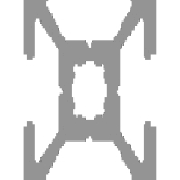
# Autodesk Inventor part: 20x20_bosch profile
Saved by Autodesk Inventor 2021.3 (Build 253353000, 353)
## iProperties
Created: 2024-01-11
Part Number: 20x20_bosch profile
Material: Aluminum 6061
Document SubType Name: Modeling
Designer: nxf77172
Language: en-US
Size Designation: (Unnamed 1)
Categories: <MemberInstance><Categories><Category DisplayName="Structural Shapes" InternalName="089c4875-fa83-4c05-b084-43b9cc11f5ed" Mnemonic="GRDR"><CategoryParameter DisplayName="Mass per Length Unit" InternalName="0bb95a10-148f-4027-a459-38d7b056702a" Mnemonic="shpmass"/><CategoryParameter DisplayName="Section Area" InternalName="1ff91680-64b0-4202-b9a3-7fd3f94bba3b" Mnemonic="secarea"/><CategoryParameter DisplayName="Radius of Gyration (x)" InternalName="25778675-03e9-40c1-b6a8-4a9ed693320d" Mnemonic="gyrradx"/><CategoryParameter DisplayName="Torsional Rigidity Modulus" InternalName="26c1ec35-5026-4c63-ad0a-751cf684a536" Mnemonic="torrigmod"/><CategoryParameter DisplayName="Distance of the Center of Gravity X-X" InternalName="26c9bdb8-9c79-4b4f-a92e-8e197583c9c4" Mnemonic="grcendistX"/><CategoryParameter DisplayName="Legacy Member ID" InternalName="340afe4f-75d7-48d3-ab7d-943f3c3da468" Mnemonic="LegacyMemberID"/><CategoryParameter DisplayName="Base Length" InternalName="42e34263-8f20-4d0e-ad48-bf1385b87c24" Mnemonic="shplen"/><CategoryParameter DisplayName="Moment of Inertia (y)" InternalName="4b9f58ea-bced-460e-81ea-3d29ca5a49e3" Mnemonic="inermomy"/><CategoryParameter DisplayName="Moment of Inertia (x)" InternalName="4cd780bc-73d7-43ac-917a-579e5cbd684d" Mnemonic="inermomx"/><CategoryParameter DisplayName="Custom Base Point" InternalName="4f1d1b73-316d-484b-a3df-9cbabb16eb77" Mnemonic="shpBasePoint"/><CategoryParameter DisplayName="Shape Height" InternalName="50274e7d-5ac0-4796-92cb-c59e54983c67" Mnemonic="shpheig"/><CategoryParameter DisplayName="Section Module (y)" InternalName="59eaa5e9-d227-48dc-b6c1-6920f96e0f95" Mnemonic="secmody"/><CategoryParameter DisplayName="Section Designation" InternalName="5a64d034-428d-49c8-ba32-7619764de20f" Mnemonic="shpdes"/><CategoryParameter DisplayName="Section Module (x)" InternalName="72cfad18-cf51-4ed4-aaa7-c6b224f8419f" Mnemonic="secmodx"/><CategoryParameter DisplayName="Torsional Section Modulus" InternalName="7c55a8dc-8844-49f9-a867-cc677b30ec9a" Mnemonic="torsecmod"/><CategoryParameter DisplayName="Shape Width" InternalName="7c717d54-a18f-4666-b4d4-573cce22c62c" Mnemonic="shpwdth"/><CategoryParameter DisplayName="Second Shape Thickness" InternalName="9251a8e1-85fd-4e47-af99-afdb762317d9" Mnemonic="shpthick2"/><CategoryParameter DisplayName="FG Authored" InternalName="9c666724-f362-4ea7-ac62-f6a007de5c69" Mnemonic="shpFGAuto"/><CategoryParameter DisplayName="Distance of the Center of Gravity Y-Y" InternalName="bcc4fb17-7af4-436a-8f8c-d0aa3b0248c5" Mnemonic="grcendistY"/><CategoryParameter DisplayName="Radius of Gyration (y)" InternalName="bfa18ebe-1636-4dbe-8d42-b263e0b73184" Mnemonic="gyrrady"/><CategoryParameter DisplayName="Shape Thickness" InternalName="d109cf76-8eb4-42fc-9800-4409734adc67" Mnemonic="shpthick"/><CategoryParameter DisplayName="Coefficient of Shear Displacement" InternalName="de4c90c6-aaa8-468f-a335-6737b311b5d3" Mnemonic="shdispc"/><Category DisplayName="Other" InternalName="f02205ff-2390-476f-921c-0b3185f88e84" Mnemonic="OTHSHP"><CategoryParameter DisplayName="Moment of Inertia (y)" InternalName="044c654e-f649-48ac-84cc-650a29ae31ca" Mnemonic="inermomy"/><CategoryParameter DisplayName="Shape Thickness" InternalName="12b1a788-9233-48fd-a933-2df8ff42b15f" Mnemonic="shpthick"/><CategoryParameter DisplayName="Mass per Length Unit" InternalName="2fd289d6-9394-4d2d-97e6-6659d7d4551d" Mnemonic="shpmass"/><CategoryParameter DisplayName="Radius of Gyration (y)" InternalName="743e1dfe-1bba-408b-b985-cf752b207386" Mnemonic="gyrrady"/><CategoryParameter DisplayName="Section Module (y)" InternalName="88b8bff9-a616-4028-93d5-ed4f79680d13" Mnemonic="secmody"/><CategoryParameter DisplayName="Section Area" InternalName="c46ecdf8-b6eb-4db9-8b25-30258930c1e3" Mnemonic="secarea"/><CategoryParameter DisplayName="Section Module (x)" InternalName="cac70804-9d39-43bb-be17-56ea1f39a6c2" Mnemonic="secmodx"/><CategoryParameter DisplayName="Moment of Inertia (x)" InternalName="ec6737bc-264f-43ed-b0bd-f6d410c2718d" Mnemonic="inermomx"/><CategoryParameter DisplayName="Radius of Gyration (x)" InternalName="ee72c61e-565e-4fd6-b448-66e1e1abcb7e" Mnemonic="gyrradx"/></Category></Category><Category DisplayName="DataType" InternalName="23b78d0f-2648-40c6-8793-ca6db495c9e8" Mnemonic="DATATYPE"><CategoryParameter DisplayName="DisplayName" InternalName="05415f3d-3907-474b-a020-eb9d644f4cf3" Mnemonic="DISPLAYNAME"/><CategoryParameter DisplayName="Standard" InternalName="0c0a119c-1e12-4c84-803f-101930972f5e" Mnemonic="STANDARD"/><CategoryParameter DisplayName="Description" InternalName="13903e3d-64b1-4950-80da-f627842ea37f" Mnemonic="DESCRIPTION"/><CategoryParameter DisplayName="Designation" InternalName="2675968c-4ce5-49e0-a4f5-552d29089031" Mnemonic="DESIGNATION"/><CategoryParameter DisplayName="Default Row" InternalName="2af9ec52-faaa-4026-b378-f9fa4afca842" Mnemonic="DEFAULTROW"/><CategoryParameter DisplayName="Folder Name" InternalName="3f06958e-8713-4116-9be7-ed6184ecc97b" Mnemonic="FOLDERNAME"/><CategoryParameter DisplayName="Revision Guid" InternalName="45a75005-10b1-4dfc-8d6d-dfe629f0b93c" Mnemonic="REVISIONGUID"/><CategoryParameter DisplayName="FileName" InternalName="8b46a4cc-9585-4fed-90c3-899f57e09a73" Mnemonic="FILENAME"/><CategoryParameter DisplayName="StdsOrg" InternalName="8f5914e1-4693-403f-8ab5-d37768198c9d" Mnemonic="STDSORG"/><CategoryParameter DisplayName="Family Version" InternalName="914462f6-6e19-4b14-ba84-155b9680b1d0" Mnemonic="FAMILYREVISION"/><CategoryParameter DisplayName="Standard Revision" InternalName="91d5a463-65c2-4fde-b823-3b7fea5e8e17" Mnemonic="STANDARDREVISION"/><CategoryParameter DisplayName="Member Revision" InternalName="a65d44b9-392f-4f4f-857b-e4b3d54996fe" Mnemonic="MEMBERREVISION"/><CategoryParameter DisplayName="ClipFormat" InternalName="bc51e27b-3422-4e78-93ef-cec197ddf230" Mnemonic="CLIPFORMAT"/><CategoryParameter DisplayName="Manufacturer" InternalName="cd6c7a72-a28a-4e50-99a9-2c7f4e13e5ad" Mnemonic="MANUFACTURER"/><CategoryParameter DisplayName="InternalName" InternalName="cf1d0246-76d9-4b4a-8305-fa0409afb5c1" Mnemonic="INTERNALNAME"/><CategoryParameter DisplayName="IsMetric" InternalName="e2385c5b-1ea4-4823-96a8-8de651266ec3" Mnemonic="ISMETRIC"/><Category DisplayName="Part" InternalName="c0e0b642-3bcb-4cc8-9e80-f96d35c4afa4" Mnemonic="PART"><CategoryParameter DisplayName="Part Number" InternalName="016b6077-bfbe-49bd-92c9-d8d59c39c941" Mnemonic="PARTNUMBER"/><CategoryParameter DisplayName="Stock Number" InternalName="4dba7c1c-e26c-444e-836c-b08b433409a8" Mnemonic="STOCKNUMBER"/><CategoryParameter DisplayName="Material Key" InternalName="5c9a8adb-dd2b-4535-b97f-0a94a95fe41f" Mnemonic="MATERIALKEY"/><CategoryParameter DisplayName="Material" InternalName="818a152a-d3c3-49ca-80ee-df7d91421b8e" Mnemonic="MATERIAL"/></Category></Category></Categories><FamilyTemplate Id="20x20_bosch profile"><FamilyTemplateParameters><FamilyTemplateParameter ObjectType="kUserParameterObject" ValueType="xs:double" Id="12" ObjectReferenceKey="Length"/><FamilyTemplateParameter ObjectType="kPartComponentDefinitionObject" ValueType="xs:string" Id="23" SubObjectId="Material"/><FamilyTemplateParameter ObjectType="kPropertyObject" ValueType="xs:string" Id="26" ObjectReferenceKey="{32853F0F-3444-11d1-9E93-0060B03C1CA6}" SubObjectId="5"/><FamilyTemplateParameter ObjectType="kPropertyObject" ValueType="xs:string" Id="27" ObjectReferenceKey="{32853F0F-3444-11d1-9E93-0060B03C1CA6}" SubObjectId="52"/></FamilyTemplateParameters></FamilyTemplate><CategoryParameterMap><ParamToTemplateMap><ParamToTemplate CategoryParameter="//CategoryParameter[@InternalName='cf1d0246-76d9-4b4a-8305-fa0409afb5c1']" ConstantValue="27b4ad4a-2417-46ba-b811-a387dd64a500"/><ParamToTemplate CategoryParameter="//CategoryParameter[@InternalName='45a75005-10b1-4dfc-8d6d-dfe629f0b93c']" ConstantValue="f0b9e895-ce42-4fe4-8826-9398c456ece3"/><ParamToTemplate CategoryParameter="//CategoryParameter[@InternalName='3f06958e-8713-4116-9be7-ed6184ecc97b']" ConstantValue="20x20_bosch profile"/><ParamToTemplate CategoryParameter="//CategoryParameter[@InternalName='8f5914e1-4693-403f-8ab5-d37768198c9d']" TemplateParameter="17"/><ParamToTemplate CategoryParameter="//CategoryParameter[@InternalName='0c0a119c-1e12-4c84-803f-101930972f5e']" TemplateParameter="18"/><ParamToTemplate CategoryParameter="//CategoryParameter[@InternalName='91d5a463-65c2-4fde-b823-3b7fea5e8e17']" TemplateParameter="19"/><ParamToTemplate CategoryParameter="//CategoryParameter[@InternalName='cd6c7a72-a28a-4e50-99a9-2c7f4e13e5ad']" TemplateParameter="20"/><ParamToTemplate CategoryParameter="//CategoryParameter[@InternalName='13903e3d-64b1-4950-80da-f627842ea37f']" TemplateParameter="22"/><ParamToTemplate CategoryParameter="//CategoryParameter[@InternalName='05415f3d-3907-474b-a020-eb9d644f4cf3']" ConstantValue="20x20_bosch profile"/><ParamToTemplate CategoryParameter="//CategoryParameter[@InternalName='914462f6-6e19-4b14-ba84-155b9680b1d0']" ConstantValue="11"/><ParamToTemplate CategoryParameter="//CategoryParameter[@InternalName='bc51e27b-3422-4e78-93ef-cec197ddf230']" ConstantValue="CF_INVENTOR.STDPARTS"/><ParamToTemplate CategoryParameter="//CategoryParameter[@InternalName='e2385c5b-1ea4-4823-96a8-8de651266ec3']" ConstantValue="true"/><ParamToTemplate CategoryParameter="//CategoryParameter[@InternalName='2af9ec52-faaa-4026-b378-f9fa4afca842']" ConstantValue="1"/><ParamToTemplate CategoryParameter="//CategoryParameter[@InternalName='9c666724-f362-4ea7-ac62-f6a007de5c69']" ConstantValue="1"/><ParamToTemplate CategoryParameter="//CategoryParameter[@InternalName='8b46a4cc-9585-4fed-90c3-899f57e09a73']" ConstantValue="Aluminum 6061-1"/><ParamToTemplate CategoryParameter="//CategoryParameter[@InternalName='a65d44b9-392f-4f4f-857b-e4b3d54996fe']" ConstantValue="857d2c95-77cc-4b79-b9be-8e574b0f7ae4"/><ParamToTemplate CategoryParameter="//CategoryParameter[@InternalName='a65d44b9-392f-4f4f-857b-e4b3d54996fe']" ConstantValue="857d2c95-77cc-4b79-b9be-8e574b0f7ae4"/><ParamToTemplate CategoryParameter="//CategoryParameter[@InternalName='2675968c-4ce5-49e0-a4f5-552d29089031']" TemplateParameter="27"/><ParamToTemplate CategoryParameter="//CategoryParameter[@InternalName='42e34263-8f20-4d0e-ad48-bf1385b87c24']" TemplateParameter="12"/><ParamToTemplate CategoryParameter="//CategoryParameter[@InternalName='818a152a-d3c3-49ca-80ee-df7d91421b8e']" TemplateParameter="23"/><ParamToTemplate CategoryParameter="//CategoryParameter[@InternalName='016b6077-bfbe-49bd-92c9-d8d59c39c941']" TemplateParameter="26"/></ParamToTemplateMap></CategoryParameterMap></MemberInstance>
Mass: 0.435942 g
Surface Area: 5.07764 cm^2
Volume: 0.16146 cm^3
Density: 2.7 g/cm^3
Appearance: Aluminum - Flat
IsCustomPart: 1
Length: 200.000 mm
G_L: 200.000 mm
G_W: 20.000 mm
G_H: 20.000 mm
_CCFamilyDisplayName: 20x20_bosch profile
_FrameMemberDoc: Frame Member File
_Version: 15.0.0
_GetPNFromCC: 1
Author: nxf77172
Autodesk Inventor part; units mm, degrees
ref_plane "YZ Plane" through (0, 0, 0) normal (1, 0, 0) x (0, 1, 0)
ref_plane "Start Plane" through (0, 0, 0) normal (0, 1, 0) x (-1, 0, 0)
ref_plane "End Plane" through (0, 200, 0) normal (0, 1, 0) x (-1, 0, 0)
sketch "Sketch" plane through (0, 0, 0) normal (0, 1, 0) x (-1, 0, 0)
  line L0 (8.5, 10) -> (3.5, 10)
  line L1 (4.5, 0.5) -> (4.5, 3.2322)
  line L2 (3.2322, 4.5) -> (0.5, 4.5)
  line L3 (3, 9.5) -> (3, 9)
  line L4 (3.5, 8.5) -> (6.2322, 8.5)
  line L5 (8.5, 6.2322) -> (8.5, 3.5)
  line L6 (9, 3) -> (9.5, 3)
  line L7 (6.5858, 7.6464) -> (3.5858, 4.6464)
  line L8 (7.6464, 6.5858) -> (4.6464, 3.5858)
  line L9 (10, 10) -> (0, 0) construction
  line L10 (0.5, 4.5) -> (0, 4)
  line L11 (3, 9.5) -> (3.5, 9.5)
  line L12 (3.5, 9.5) -> (3.5, 10)
  line L13 (9.5, 3) -> (9.5, 3.5)
  line L14 (9.5, 3.5) -> (10, 3.5)
  line L15 (10, 3.5) -> (10, 10)
  line L16 (0, 0) -> (10, 0) construction
  line L17 (10, 0) -> (10, 8.5) construction
  line L18 (0, 0) -> (0, 10) construction
  line L19 (0, 10) -> (10, 10) construction
  line L20 (4.5, 0.5) -> (4, 0)
  arc A0 (10, 8.5) -> (8.5, 10) centre (8.5, 8.5) ccw
  arc A1 (3, 9) -> (3.5, 8.5) centre (3.5, 9) ccw
  arc A2 (6.5858, 7.6464) -> (6.2322, 8.5) centre (6.2322, 8) ccw
  arc A3 (8.5, 6.2322) -> (7.6464, 6.5858) centre (8, 6.2322) ccw
  arc A4 (8.5, 3.5) -> (9, 3) centre (9, 3.5) ccw
  arc A5 (4.6464, 3.5858) -> (4.5, 3.2322) centre (5, 3.2322) ccw
  arc A6 (3.2322, 4.5) -> (3.5858, 4.6464) centre (3.2322, 5) ccw
  line L21 (2.2657, 2.2657) -> (1.9121, 2.6192)
  line L22 (2.2657, 2.2657) -> (2.6192, 1.9121)
  line L23 (1.9121, 2.6192) -> (1.5586, 2.2657)
  line L24 (2.6192, 1.9121) -> (2.2657, 1.5586)
  arc A7 (2.75, 0) -> (2.2657, 1.5586) centre (0, 0) ccw
  arc A8 (1.5586, 2.2657) -> (0, 2.75) centre (0, 0) ccw
  line L25 (0, 0) -> (10, 0) construction
  line L26 (10, -10) -> (0, 0) construction
  line L27 (0, 0) -> (0, -10) construction
  line L28 (0, -10) -> (8.5, -10) construction
  line L29 (0.5, -4.5) -> (3.2322, -4.5)
  line L30 (0.5, -4.5) -> (0, -4)
  line L31 (1.9121, -2.6192) -> (1.5586, -2.2657)
  arc A9 (0, -2.75) -> (1.5586, -2.2657) centre (0, 0) ccw
  arc A10 (7.6464, -6.5858) -> (8.5, -6.2322) centre (8, -6.2322) ccw
  line L32 (8.5, -3.5) -> (8.5, -6.2322)
  line L33 (10, -8.5) -> (10, -3.5)
  line L34 (3.5, -10) -> (10, -10)
  line L35 (6.5858, -7.6464) -> (3.5858, -4.6464)
  line L36 (7.6464, -6.5858) -> (4.6464, -3.5858)
  line L37 (10, 0) -> (10, -10) construction
  line L38 (4.5, -3.2322) -> (4.5, -0.5)
  arc A11 (8.5, -10) -> (10, -8.5) centre (8.5, -8.5) ccw
  line L39 (6.2322, -8.5) -> (3.5, -8.5)
  arc A12 (3.5, -8.5) -> (3, -9) centre (3.5, -9) ccw
  arc A13 (6.2322, -8.5) -> (6.5858, -7.6464) centre (6.2322, -8) ccw
  line L40 (3, -9.5) -> (3.5, -9.5)
  line L41 (3.5, -9.5) -> (3.5, -10)
  line L42 (9.5, -3) -> (9, -3)
  line L43 (4.5, -0.5) -> (4, 0)
  line L44 (9.5, -3) -> (9.5, -3.5)
  line L45 (9.5, -3.5) -> (10, -3.5)
  arc A14 (4.5, -3.2322) -> (4.6464, -3.5858) centre (5, -3.2322) ccw
  arc A15 (9, -3) -> (8.5, -3.5) centre (9, -3.5) ccw
  arc A16 (3.5858, -4.6464) -> (3.2322, -4.5) centre (3.2322, -5) ccw
  line L46 (3, -9) -> (3, -9.5)
  line L47 (2.2657, -2.2657) -> (2.6192, -1.9121)
  line L48 (2.2657, -2.2657) -> (1.9121, -2.6192)
  line L49 (2.6192, -1.9121) -> (2.2657, -1.5586)
  arc A17 (2.2657, -1.5586) -> (2.75, 0) centre (0, 0) ccw
  line L50 (0, 0) -> (0, -10) construction
  line L51 (-10, -10) -> (0, 0) construction
  line L52 (0, 0) -> (-10, 0) construction
  line L53 (-10, 0) -> (-10, -8.5) construction
  line L54 (-4.5, -0.5) -> (-4.5, -3.2322)
  line L55 (-4.5, -0.5) -> (-4, 0)
  line L56 (-2.6192, -1.9121) -> (-2.2657, -1.5586)
  arc A18 (-2.75, 0) -> (-2.2657, -1.5586) centre (0, 0) ccw
  arc A19 (-6.5858, -7.6464) -> (-6.2322, -8.5) centre (-6.2322, -8) ccw
  line L57 (-3.5, -8.5) -> (-6.2322, -8.5)
  line L58 (-8.5, -10) -> (-3.5, -10)
  line L59 (-10, -3.5) -> (-10, -10)
  line L60 (-7.6464, -6.5858) -> (-4.6464, -3.5858)
  line L61 (-6.5858, -7.6464) -> (-3.5858, -4.6464)
  line L62 (0, -10) -> (-10, -10) construction
  line L63 (-3.2322, -4.5) -> (-0.5, -4.5)
  arc A20 (-10, -8.5) -> (-8.5, -10) centre (-8.5, -8.5) ccw
  line L64 (-8.5, -6.2322) -> (-8.5, -3.5)
  arc A21 (-8.5, -3.5) -> (-9, -3) centre (-9, -3.5) ccw
  arc A22 (-8.5, -6.2322) -> (-7.6464, -6.5858) centre (-8, -6.2322) ccw
  line L65 (-9.5, -3) -> (-9.5, -3.5)
  line L66 (-9.5, -3.5) -> (-10, -3.5)
  line L67 (-3, -9.5) -> (-3, -9)
  line L68 (-0.5, -4.5) -> (0, -4)
  line L69 (-3, -9.5) -> (-3.5, -9.5)
  line L70 (-3.5, -9.5) -> (-3.5, -10)
  arc A23 (-3.2322, -4.5) -> (-3.5858, -4.6464) centre (-3.2322, -5) ccw
  arc A24 (-3, -9) -> (-3.5, -8.5) centre (-3.5, -9) ccw
  arc A25 (-4.6464, -3.5858) -> (-4.5, -3.2322) centre (-5, -3.2322) ccw
  line L71 (-9, -3) -> (-9.5, -3)
  line L72 (-2.2657, -2.2657) -> (-1.9121, -2.6192)
  line L73 (-2.2657, -2.2657) -> (-2.6192, -1.9121)
  line L74 (-1.9121, -2.6192) -> (-1.5586, -2.2657)
  arc A26 (-1.5586, -2.2657) -> (0, -2.75) centre (0, 0) ccw
  line L75 (0, 0) -> (-10, 0) construction
  line L76 (-10, 10) -> (0, 0) construction
  line L77 (0, 0) -> (0, 10) construction
  line L78 (0, 10) -> (-8.5, 10) construction
  line L79 (-0.5, 4.5) -> (-3.2322, 4.5)
  line L80 (-0.5, 4.5) -> (0, 4)
  line L81 (-1.9121, 2.6192) -> (-1.5586, 2.2657)
  arc A27 (0, 2.75) -> (-1.5586, 2.2657) centre (0, 0) ccw
  arc A28 (-7.6464, 6.5858) -> (-8.5, 6.2322) centre (-8, 6.2322) ccw
  line L82 (-8.5, 3.5) -> (-8.5, 6.2322)
  line L83 (-10, 8.5) -> (-10, 3.5)
  line L84 (-3.5, 10) -> (-10, 10)
  line L85 (-6.5858, 7.6464) -> (-3.5858, 4.6464)
  line L86 (-7.6464, 6.5858) -> (-4.6464, 3.5858)
  line L87 (-10, 0) -> (-10, 10) construction
  line L88 (-4.5, 3.2322) -> (-4.5, 0.5)
  arc A29 (-8.5, 10) -> (-10, 8.5) centre (-8.5, 8.5) ccw
  line L89 (-6.2322, 8.5) -> (-3.5, 8.5)
  arc A30 (-3.5, 8.5) -> (-3, 9) centre (-3.5, 9) ccw
  arc A31 (-6.2322, 8.5) -> (-6.5858, 7.6464) centre (-6.2322, 8) ccw
  line L90 (-3, 9.5) -> (-3.5, 9.5)
  line L91 (-3.5, 9.5) -> (-3.5, 10)
  line L92 (-9.5, 3) -> (-9, 3)
  line L93 (-4.5, 0.5) -> (-4, 0)
  line L94 (-9.5, 3) -> (-9.5, 3.5)
  line L95 (-9.5, 3.5) -> (-10, 3.5)
  arc A32 (-4.5, 3.2322) -> (-4.6464, 3.5858) centre (-5, 3.2322) ccw
  arc A33 (-9, 3) -> (-8.5, 3.5) centre (-9, 3.5) ccw
  arc A34 (-3.5858, 4.6464) -> (-3.2322, 4.5) centre (-3.2322, 5) ccw
  line L96 (-3, 9) -> (-3, 9.5)
  line L97 (-2.2657, 2.2657) -> (-2.6192, 1.9121)
  line L98 (-2.2657, 2.2657) -> (-1.9121, 2.6192)
  line L99 (-2.6192, 1.9121) -> (-2.2657, 1.5586)
  arc A35 (-2.2657, 1.5586) -> (-2.75, 0) centre (0, 0) ccw
  point P0 (0, 2.75)
  point P1 (-4, 0)
  point P2 (0, -4)
  dimension "d4" = 5.5
  dimension "d5" = 1.5
  dimension "d9" = 1.5
  dimension "d13" = 0.5
  dimension "d14" = 0.5
  dimension "d21" = 0.5
  dimension "d22" = 0.5
  dimension "d23" = 0.5
  dimension "d25" = 1.5
  dimension "d26" = 10
  dimension "d27" = 10
  dimension "d28" = 3
  dimension "d29" = 3
  dimension "d30" = 5.5
  dimension "d31" = 1.5
  dimension "d32" = 0.5
  dimension "d33" = 0.5
  dimension "d34" = 0.5
  dimension "d35" = 0.5
  dimension "d36" = 0.5
  dimension "d37" = 0.5
  dimension "d38" = 0.5
  dimension "d39" = 0.5
  dimension "d40" = 0.5
  dimension "d41" = 2.75
  dimension "d42" = 2.75
  dimension "d43" = 0.5
  dimension "d46" = 360
  constraints: 200 end point, 72 point on circle, 36 centre point, 28 point on line, 14 perpendicular, 14 tangent, 10 coincident, 2 parallel, 2 vertical, 1 collinear, 312 other
  measures "d4" distance between parallel lines of L0 L2
  measures "d5" distance between parallel lines of L0 L4
  measures "d9" distance between parallel lines of L8 L7
  measures "d13" distance from line of L10.end L2
  measures "d14" distance of L6.end L13.end
  measures "d21" distance from line of L16 L1.start
  measures "d22" distance from line of L1 L20.end
  measures "d23" distance from line of L18 L2.end
  measures "d25" distance between parallel lines of L5 L15
  measures "d26" distance between parallel lines of L16 L0
  measures "d27" distance between parallel lines of L18 L17
  measures "d28" distance between parallel lines of L6 L16
  measures "d29" distance between parallel lines of L18 L3
  measures "d30" distance between parallel lines of L15 L1
  measures "d31" radius of A0
  measures "d32" radius of A1
  measures "d33" radius of A2
  measures "d34" radius of A3
  measures "d35" radius of A4
  measures "d36" radius of A5
  measures "d37" radius of A6
  measures "d38" distance from line of L22.end L9
  measures "d39" distance from line of L21.end L9
  measures "d40" distance of L21.end L23.end
  measures "d41" radius of A8
  measures "d42" radius of A7
  measures "d43" distance of L22.end L24.end
extrude "Body" add sketch "Sketch" along normal up to surface (200 mm away) from surface at 0
sketch "Sketch2" plane through (0, 0, 0) normal (0, 1, 0) x (-1, 0, 0)
  line L0 (0, 0) -> (10, 0)
ref_plane "Work Plane3" through (0, 0, 0) normal (0, 0, -1) x (-1, 0, 0)
sketch "Sketch3" plane through (0, 0, 0) normal (0, 0, -1) x (-1, 0, 0)
  line L0 (-2, 0) -> (12, 0)
  line L1 (-2, 200) -> (12, 200)
  dimension "d55" = 200
  measures "d55" distance between parallel lines of L0 L1
equation "\"d4\" = d30"
equation "\"d13\" = d21"
equation "\"d22\" = d21"
equation "\"d23\" = d21"
equation "\"d25\" = d5"
equation "\"d29\" = d28"
equation "\"d39\" = d38"
equation "\"d42\" = d41"
equation "\"d43\" = d40"
equation "\"d6\" = d5"
equation "\"Length\" = 200"
equation "\"G_OFFSET_START\" = 0"
equation "\"G_OFFSET_END\" = 0"
equation "\"G_L\" = d55"
